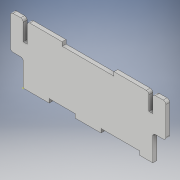
# Autodesk Inventor part: front_left_v2
Saved by Autodesk Inventor 2017.2 (Build 212233000, 233)
## iProperties
Created: 2017-06-09
Part Number: front_left_v2
Material: Generic
Document SubType Name: Modeling
Designer: SandeepSH
Density: 1 g/cm^3
Appearance: Default
Author: SandeepSH
Autodesk Inventor part; units mm, degrees
ref_plane "YZ Plane" through (0, 0, 0) normal (1, 0, 0) x (0, 1, 0)
ref_plane "XZ Plane" through (0, 0, 0) normal (0, 1, 0) x (-1, 0, 0)
ref_plane "XY Plane" through (0, 0, 0) normal (0, 0, 1) x (1, 0, 0)
sketch "Sketch1" plane through (0, 0, 0) normal (0, 0, 1) x (1, 0, 0)
  line L0 (0, 0) -> (100, 0)
  line L1 (100, 0) -> (100, 46)
  line L2 (100, 46) -> (0, 46)
  line L3 (0, 46) -> (0, 0)
  dimension "d0" = 100
  dimension "d1" = 46
  constraints: 8 end point, 2 parallel, 1 horizontal, 1 perpendicular
  measures "d0" distance of L2.end L1.end
  measures "d1" distance of L1.end L0.end
extrude "Extrusion1" add sketch "Sketch1" along normal blind 3
sketch "Sketch2" plane through (0, 0, 3) normal (0, 0, 1) x (1, 0, 0)
  line L0 (0, 0) -> (100, 0) projected
  line L1 (20, 0) -> (40, 0)
  line L2 (40, 0) -> (40, 3)
  line L3 (40, 3) -> (20, 3)
  line L4 (20, 3) -> (20, 0)
  line L5 (0, 46) -> (0, 0) projected
  line L6 (60, 0) -> (90, 0)
  line L7 (90, 0) -> (90, 3)
  line L8 (90, 3) -> (60, 3)
  line L9 (60, 3) -> (60, 0)
  line L10 (100, 0) -> (100, 46) projected
  line L11 (100, 46) -> (0, 46) projected
  line L12 (30, 46) -> (70, 46)
  line L13 (70, 46) -> (70, 43)
  line L14 (70, 43) -> (30, 43)
  line L15 (30, 43) -> (30, 46)
  dimension "d4" = 3
  dimension "d5" = 20
  dimension "d6" = 20
  dimension "d8" = 3
  dimension "d9" = 20
  dimension "d10" = 10
  dimension "d11" = 3
  dimension "d12" = 30
  dimension "d13" = 30
  constraints: 24 end point, 6 parallel, 3 horizontal, 3 perpendicular, 3 point on line
  measures "d4" distance of L2.end L1.end
  measures "d5" distance between parallel lines of L5 L4
  measures "d6" distance between parallel lines of L2 L4
  measures "d8" distance of L7.end L6.end
  measures "d9" distance between parallel lines of L9 L2
  measures "d10" distance between parallel lines of L10 L7
  measures "d11" distance of L12.end L13.end
  measures "d12" distance between parallel lines of L15 L5
  measures "d13" distance between parallel lines of L10 L13
extrude "Extrusion2" cut sketch "Sketch2" against normal through all contours L4 L3 L2 L0 | L11 L13 L14 L15 | L9 L8 L7 L0
sketch "Sketch3" plane through (0, 0, 3) normal (0, 0, 1) x (1, 0, 0)
  line L0 (100, 0) -> (100, 46) projected
  line L1 (100, 46) -> (97, 46)
  line L2 (97, 46) -> (97, 33)
  line L3 (97, 33) -> (100, 33)
  line L4 (100, 33) -> (100, 46)
  point P0 (0, 0)
  dimension "d16" = 3
  dimension "d17" = 13
  constraints: 8 end point, 2 parallel, 1 horizontal, 1 perpendicular
  measures "d16" distance of L3.end L2.end
  measures "d17" distance of L2.end L1.end
extrude "Extrusion3" cut sketch "Sketch3" against normal through all
sketch "Sketch4" plane through (0, 0, 3) normal (0, 0, 1) x (1, 0, 0)
  line L0 (97, 46) -> (70, 46) projected
  line L1 (100, 0) -> (100, 33) projected
  line L2 (100, 20) -> (110, 20)
  line L3 (110, 20) -> (110, 46)
  line L4 (110, 46) -> (100, 46)
  line L5 (100, 46) -> (100, 20)
  line L6 (90, 0) -> (100, 0) projected
  point P0 (0, 0)
  dimension "d20" = 10
  dimension "d21" = 20
  constraints: 8 end point, 2 parallel, 1 collinear, 1 horizontal, 1 perpendicular, 1 point on line
  measures "d20" distance of L4.end L3.end
  measures "d21" distance between parallel lines of L2 L6
extrude "Extrusion4" add sketch "Sketch4" against normal blind 3
sketch "Sketch5" plane through (0, 0, 3) normal (0, 0, 1) x (1, 0, 0)
  line L0 (0, 46) -> (0, 0) projected
  line L1 (0, 46) -> (-10, 46)
  line L2 (-10, 46) -> (-10, 20)
  line L3 (-10, 20) -> (0, 20)
  line L4 (0, 20) -> (0, 46)
  line L5 (0, 0) -> (20, 0) projected
  dimension "d24" = 10
  dimension "d25" = 20
  constraints: 8 end point, 2 parallel, 1 horizontal, 1 perpendicular
  measures "d24" distance of L3.end L2.end
  measures "d25" distance between parallel lines of L5 L3
extrude "Extrusion5" add sketch "Sketch5" against normal blind 3
sketch "Sketch6" plane through (0, 0, 3) normal (0, 0, 1) x (1, 0, 0)
  point P0 (0, 0)
sketch "Sketch7" plane through (0, 0, 3) normal (0, 0, 1) x (1, 0, 0)
  line L0 (30, 46) -> (-10, 46) projected
  line L1 (0, 46) -> (3, 46)
  line L2 (3, 46) -> (3, 31)
  line L3 (3, 31) -> (0, 31)
  line L4 (0, 31) -> (0, 46)
  point P0 (0, 0)
  dimension "d28" = 3
  dimension "d29" = 15
  constraints: 8 end point, 2 parallel, 1 horizontal, 1 perpendicular, 1 point on line
  measures "d28" distance of L2.end L3.end
  measures "d29" distance of L1.end L2.end
extrude "Extrusion6" cut sketch "Sketch7" against normal through all
fillet "Fillet1" radius 2 10 edges at (0, 46, 1.5) (3, 46, 1.5) (-10, 46, 1.5) (97, 46, 1.5) (100, 46, 1.5) (110, 46, 1.5) (110, 20, 1.5) (100, 20, 1.5) (-10, 20, 1.5) (0, 20, 1.5)
equation "\"d6\" = d5"
equation "\"d9\" = d6"
body "Solid1"
